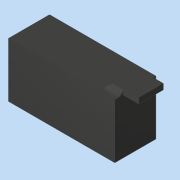
# Autodesk Inventor part: ASDSBattery
Saved by Autodesk Inventor 2020.3 (Build 243373000, 373)
## iProperties
Created: 2019-07-29
Part Number: ASDSBattery
Material: ABS Plastic
Document SubType Name: Modeling
Designer: Derek Wider
Density: 1.06 g/cm^3
Appearance: Smooth - Black
Author: Derek Wider
Autodesk Inventor part; units mm, degrees
ref_plane "YZ Plane" through (0, 0, 0) normal (1, 0, 0) x (0, 1, 0)
ref_plane "XZ Plane" through (0, 0, 0) normal (0, 1, 0) x (-1, 0, 0)
ref_plane "XY Plane" through (0, 0, 0) normal (0, 0, 1) x (1, 0, 0)
sketch "Sketch1" plane through (0, 0, 0) normal (0, 0, 1) x (1, 0, 0)
  line L0 (0, 0) -> (60.452, 0)
  line L1 (60.452, 0) -> (60.452, 30.988)
  line L2 (60.452, 30.988) -> (0, 30.988)
  line L3 (0, 30.988) -> (0, 0)
  dimension "d0" = 60.452
  dimension "d1" = 30.988
  constraints: 8 end point, 2 parallel, 1 horizontal, 1 perpendicular
  measures "d0" distance of L2.end L1.end
  measures "d1" distance of L1.end L0.end
extrude "Extrusion1" add sketch "Sketch1" along normal blind 23.368
sketch "Sketch2" plane through (60.452, 0, 0) normal (1, 0, 0) x (0, 0, -1)
  line L0 (-4.699, 30.988) -> (-18.669, 30.988)
  line L1 (-18.669, 30.988) -> (-18.669, 34.163)
  line L2 (-18.669, 34.163) -> (-4.699, 34.163)
  line L3 (-4.699, 34.163) -> (-4.699, 30.988)
  line L4 (0, 30.988) -> (-23.368, 30.988) projected
  point P0 (0, 0)
  point P1 (-11.684, 34.163)
  point P2 (-11.684, 30.988)
  point P3 (-11.684, 30.988)
  dimension "d4" = 13.97
  dimension "d5" = 3.175
  constraints: 8 end point, 3 midpoint, 2 parallel, 1 coincident, 1 horizontal, 1 perpendicular, 1 point on line, 1 vertical alignment
  measures "d4" distance of L1.end L2.end
  measures "d5" distance of L2.end L0.start
extrude "Extrusion2" add sketch "Sketch2" along normal blind 8.89 and the other way blind 6.35
fillet "Fillet1" radius 3.175 3 edges at (54.102, 30.988, 11.684) (57.277, 30.988, 18.669) (57.277, 30.988, 4.699)
body "Solid1"
